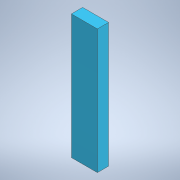
# Autodesk Inventor part: lcd2
Saved by Autodesk Inventor 2021 (Build 250183000, 183)
## iProperties
Created: 2021-07-13
Part Number: lcd2
Material: Generic
Document SubType Name: Modeling
Designer: Dell
Density: 1 g/cm^3
Appearance: Default
Author: Dell
Autodesk Inventor part; units mm, degrees
ref_plane "YZ Plane" through (0, 0, 0) normal (1, 0, 0) x (0, 1, 0)
ref_plane "XZ Plane" through (0, 0, 0) normal (0, 1, 0) x (-1, 0, 0)
ref_plane "XY Plane" through (0, 0, 0) normal (0, 0, 1) x (1, 0, 0)
sketch "Sketch1" plane through (0, 0, 0) normal (0, 0, 1) x (1, 0, 0)
  line L0 (0.5461, 8.9335) -> (2.8575, 8.9335)
  line L1 (2.8575, 8.9335) -> (2.8575, -2.1187)
  line L2 (2.8575, -2.1187) -> (0.5461, -2.1187)
  line L3 (0.5461, -2.1187) -> (0.5461, 8.9335)
  point P0 (0, 0)
  dimension "d0" = 2.3114
  constraints: 8 end point, 2 parallel, 1 horizontal, 1 perpendicular
  measures "d0" distance of L1.end L2.end
extrude "Extrusion1" add sketch "Sketch1" along normal blind 1
body "Solid1"
